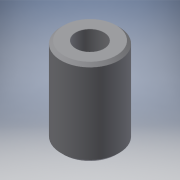
# Autodesk Inventor part: TestPart
Saved by Autodesk Inventor 2016 SP1 (Build 200210100, 210)
## iProperties
Created: 2007-04-12
Part Number: TestPart
Document SubType Name: Modeling
Designer: leefsmp
Density: 1 g/cm^3
Material: Generic
Appearance: Default
Author: leefsmp
Autodesk Inventor part; units mm, degrees
ref_plane "YZ Plane" through (0, 0, 0) normal (1, 0, 0) x (0, 1, 0)
ref_plane "XZ Plane" through (0, 0, 0) normal (0, 1, 0) x (-1, 0, 0)
ref_plane "XY Plane" through (0, 0, 0) normal (0, 0, 1) x (1, 0, 0)
sketch "Sketch1" plane through (0, 0, 0) normal (0, 0, 1) x (1, 0, 0)
  line L0 (-32.3193, 1438.8965) -> (230.2753, 1438.8965)
  line L1 (230.2753, 1438.8965) -> (230.2753, -61.1035)
  line L2 (230.2753, -61.1035) -> (-32.3193, -61.1035)
  line L3 (-32.3193, -61.1035) -> (-32.3193, 1438.8965)
  line L4 (474.8029, 1305.3567) -> (474.8029, 344.6217)
  dimension "d10" = 1500
  constraints: 10 end point, 3 parallel, 1 horizontal, 1 perpendicular
  measures "d10" distance of L2.end L0.start
revolve "Revolution1" add sketch "Sketch1" angle 360 about axis through (474.8029, 1305.3567, 0) along (0, -1, 0)
chamfer "Chamfer1" distance 3.175 angle 45 2 edges at (719.3305, 1438.8965, 0) (719.3305, -61.1035, 0)
chamfer "Chamfer3" distance 50 angle 45 2 edges at (981.9251, 1438.8965, 0) (981.9251, -61.1035, 0)
body "Solid1"
